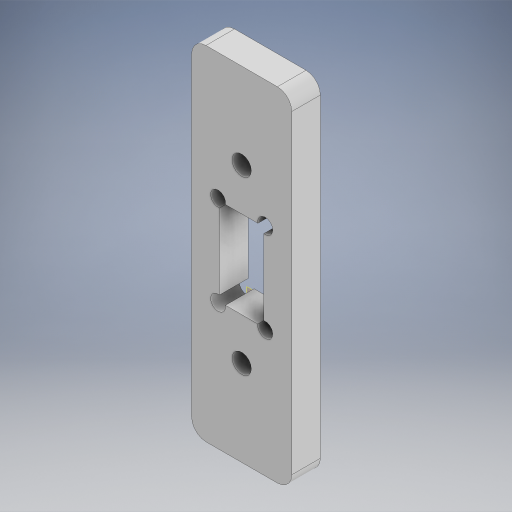
# Autodesk Inventor part: hand connection_zig1
Saved by Autodesk Inventor 2024 (Build 280153000, 153)
## iProperties
Created: 2024-09-11
Part Number: hand connection_zig1
Material: 일반
Document SubType Name: Modeling
Designer: ASUS
Density: 1 g/cm^3
Appearance: 기본값
Author: ASUS
Autodesk Inventor part; units mm, degrees
ref_plane "YZ Plane" through (0, 0, 0) normal (1, 0, 0) x (0, 1, 0)
ref_plane "XZ Plane" through (0, 0, 0) normal (0, 1, 0) x (-1, 0, 0)
ref_plane "XY Plane" through (0, 0, 0) normal (0, 0, 1) x (1, 0, 0)
ref_plane "작업 평면1" through (0, -21, 0) normal (0, 0, 1) x (1, 0, 0)
sketch "스케치1" plane through (0, -21, 0) normal (0, 0, 1) x (1, 0, 0)
  line L0 (0, 12) -> (0, 0) projected
  line L1 (0, 0) -> (6, 0) projected
  line L2 (6, 12) -> (6, 0) projected
  line L3 (0, 12) -> (6, 12) projected
  line L4 (6.3, -0.3) -> (-0.3, -0.3)
  line L5 (-0.3, -0.3) -> (-0.3, 12.3)
  line L6 (-0.3, 12.3) -> (6.3, 12.3)
  line L7 (6.3, 12.3) -> (6.3, -0.3)
  circle A0 centre (6.3, 12.3) radius 1.05
  circle A1 centre (6.3, -0.3) radius 1.05
  circle A2 centre (-0.3, 12.3) radius 1.05
  circle A3 centre (-0.3, -0.3) radius 1.05
  line L8 (0, 13) -> (6, 13) projected
  line L9 (6, 13) -> (6, 26) projected
  line L10 (0, 26) -> (6, 26) projected
  line L11 (0, 13) -> (0, 26) projected
  circle A4 centre (3, 18) radius 1.35 projected
  line L12 (6, -1) -> (0, -1) projected
  line L13 (0, -1) -> (0, -14) projected
  line L14 (6, -14) -> (0, -14) projected
  line L15 (6, -1) -> (6, -14) projected
  circle A5 centre (3, -6) radius 1.35 projected
  line L16 (6, 26) -> (0, 26)
  line L17 (0, 26) -> (0, -14)
  line L18 (0, -14) -> (6, -14)
  line L19 (6, -14) -> (6, 26)
  line L20 (10, 30) -> (-4, 30)
  line L21 (-4, 30) -> (-4, -18)
  line L22 (-4, -18) -> (10, -18)
  line L23 (10, -18) -> (10, 30)
  point P0 (0, 21)
  point P1 (0.75, 12.3)
  point P2 (5.25, 12.3)
  point P3 (6.3, 11.25)
  point P4 (6.3, 0.75)
  point P5 (5.25, -0.3)
  point P6 (0.75, -0.3)
  point P7 (-0.3, 0.75)
  point P8 (-0.3, 11.25)
  dimension "d0" = 0.3
  dimension "d1" = 2.1
  dimension "d2" = 2.1
  dimension "d3" = 2.1
  dimension "d4" = 2.1
  dimension "d5" = 4
  constraints: 24 end point, 4 centre point, 4 coincident, 4 parallel, 2 perpendicular, 1 horizontal, 6 other
  measures "d0" distance between parallel lines of L2 L7
  measures "d1" diameter of A0
  measures "d2" diameter of A1
  measures "d3" diameter of A2
  measures "d4" diameter of A3
  measures "d5" distance between parallel lines of L19 L23
extrude "돌출1" add sketch "스케치1" along normal blind 4 contours A2 L8 A0 L6 | L11 L10 L9 A0 L8 A2 | L4 A1 L12 A3 | A3 L12 A1 L15 L14 L13 | L23 L22 L21 L20
fillet "모깎기1" radius 2 4 edges at (10, 9, 2) (-4, 9, 2) (10, -39, 2) (-4, -39, 2)
sketch "스케치2" plane through (0, -21, 0) normal (0, 0, -1) x (-1, 0, 0)
  arc A0 (2, -18) -> (4, -16) centre (2, -16) ccw projected
  line L0 (4, 28) -> (4, -16) projected
  arc A1 (4, 28) -> (2, 30) centre (2, 28) ccw projected
  line L1 (-8, 30) -> (2, 30) projected
  arc A2 (-8, 30) -> (-10, 28) centre (-8, 28) ccw projected
  line L2 (-10, -16) -> (-10, 28) projected
  arc A3 (-10, -16) -> (-8, -18) centre (-8, -16) ccw projected
  line L3 (2, -18) -> (-8, -18) projected
  circle A4 centre (-3, -6) radius 1.35 projected
  circle A5 centre (-3, 18) radius 1.35 projected
  arc A6 (0.3, 11.25) -> (-0.75, 12.3) centre (0.3, 12.3) ccw projected
  line L4 (0.3, 0.75) -> (0.3, 11.25) projected
  arc A7 (-0.75, -0.3) -> (0.3, 0.75) centre (0.3, -0.3) ccw projected
  line L5 (-5.25, -0.3) -> (-0.75, -0.3) projected
  arc A8 (-6.3, 0.75) -> (-5.25, -0.3) centre (-6.3, -0.3) ccw projected
  line L6 (-6.3, 11.25) -> (-6.3, 0.75) projected
  arc A9 (-5.25, 12.3) -> (-6.3, 11.25) centre (-6.3, 12.3) ccw projected
  line L7 (-0.75, 12.3) -> (-5.25, 12.3) projected
  arc A10 (-0.5261, -0.1) -> (0.1, 0.5261) centre (0.3, -0.3) ccw
  line L8 (0.1, 0.5261) -> (0.1, 11.4739)
  arc A11 (0.1, 11.4739) -> (-0.5261, 12.1) centre (0.3, 12.3) ccw
  line L9 (-0.5261, 12.1) -> (-5.4739, 12.1)
  arc A12 (-5.4739, 12.1) -> (-6.1, 11.4739) centre (-6.3, 12.3) ccw
  line L10 (-6.1, 11.4739) -> (-6.1, 0.5261)
  arc A13 (-6.1, 0.5261) -> (-5.4739, -0.1) centre (-6.3, -0.3) ccw
  line L11 (-5.4739, -0.1) -> (-0.5261, -0.1)
  point P0 (0, 21)
  dimension "d9" = 0.2
  constraints: 8 end point, 8 point on circle, 4 centre point, 7 other
  measures "d9" distance between parallel lines of L5 L11
extrude "돌출2" add sketch "스케치2" against normal up to surface (4 mm away) contours L4 A7 L5 A8 L6 A9 L7 A6
sketch "스케치3" plane through (0, -21, 4) normal (0, 0, 1) x (1, 0, 0)
  arc A0 (5.4739, -0.1) -> (6.1, 0.5261) centre (6.3, -0.3) ccw projected
  line L0 (0.5261, -0.1) -> (5.4739, -0.1) projected
  arc A1 (-0.1, 0.5261) -> (0.5261, -0.1) centre (-0.3, -0.3) ccw projected
  line L1 (-0.1, 11.4739) -> (-0.1, 0.5261) projected
  arc A2 (0.5261, 12.1) -> (-0.1, 11.4739) centre (-0.3, 12.3) ccw projected
  line L2 (5.4739, 12.1) -> (0.5261, 12.1) projected
  arc A3 (6.1, 11.4739) -> (5.4739, 12.1) centre (6.3, 12.3) ccw projected
  line L3 (6.1, 0.5261) -> (6.1, 11.4739) projected
  arc A4 (-4, -16) -> (-2, -18) centre (-2, -16) ccw projected
  line L4 (-2, -18) -> (8, -18) projected
  arc A5 (8, -18) -> (10, -16) centre (8, -16) ccw projected
  line L5 (10, -16) -> (10, 28) projected
  arc A6 (10, 28) -> (8, 30) centre (8, 28) ccw projected
  line L6 (8, 30) -> (-2, 30) projected
  arc A7 (-2, 30) -> (-4, 28) centre (-2, 28) ccw projected
  line L7 (-4, 28) -> (-4, -16) projected
  circle A8 centre (3, -6) radius 1.35 projected
  circle A9 centre (3, 18) radius 1.35 projected
  point P0 (0, 21)
hole "구멍1" at (6.3, -8.7, 4) at (-0.3, -8.7, 4) at (6.3, -21.3, 4) at (-0.3, -21.3, 4) direction (0, 0, -1) diameter 2.1 end through all
